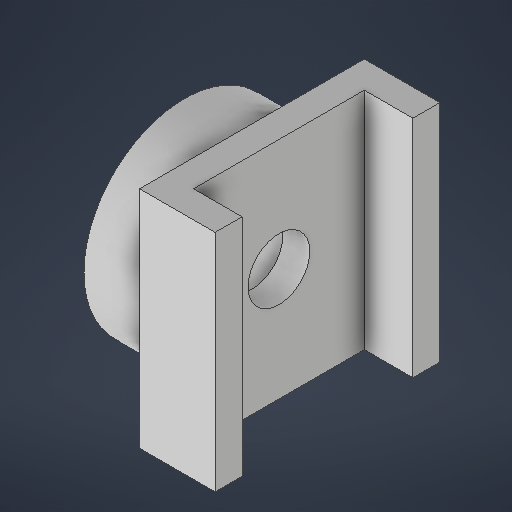
# Autodesk Inventor part: MMAE 232 CAD Assignment 2 Servo Horn 2-Nicholas Skiba
Saved by Autodesk Inventor 2026.1 (Build 301233000, 233)
## iProperties
Created: 2025-08-27
Part Number: MMAE 232 CAD Assignment 2 Servo Horn 2-Nicholas Skiba
Material: Generic
Document SubType Name: Modeling
Designer: Nick
Density: 1 g/cm^3
Appearance: Default
Author: Nick
Autodesk Inventor part; units mm, degrees
ref_plane "YZ Plane" through (0, 0, 0) normal (1, 0, 0) x (0, 1, 0)
ref_plane "XZ Plane" through (0, 0, 0) normal (0, 1, 0) x (-1, 0, 0)
ref_plane "XY Plane" through (0, 0, 0) normal (0, 0, 1) x (1, 0, 0)
sketch "Sketch1" plane through (0, 0, 0) normal (0, 1, 0) x (-1, 0, 0)
  line L0 (0, 0) -> (3.36, 0)
  line L1 (3.36, 0) -> (3.36, -10)
  line L2 (3.36, -10) -> (0, -10)
  line L3 (0, -10) -> (0, -8.8)
  line L4 (0, -8.8) -> (2.16, -8.8)
  line L5 (2.16, -8.8) -> (2.16, -1.2)
  line L6 (2.16, -1.2) -> (0, -1.2)
  line L7 (0, -1.2) -> (0, 0)
  dimension "d0" = 3.36
  dimension "d1" = 10
  dimension "d2" = 1.2
  dimension "d3" = 2.16
  dimension "d4" = 7.6
  constraints: 16 end point, 6 perpendicular, 1 horizontal, 1 point on line, 1 vertical
  measures "d0" distance of L0.start L0.end
  measures "d1" distance of L0.end L1.end
  measures "d2" distance of L2.end L3.end
  measures "d3" distance of L3.end L4.end
  measures "d4" distance of L4.end L5.end
extrude "Extrusion1" add sketch "Sketch1" along normal blind 10
sketch "Sketch2" plane through (-3.36, 0, -10) normal (-1, 0, 0) x (0, 0, 1)
  line L0 (1.2, 0) -> (0, 0) projected
  line L1 (0, 0) -> (0, 5)
  line L2 (0, 5) -> (5, 5)
  circle A0 centre (5, 5) radius 1.37
  circle A1 centre (5, 5) radius 2.75
  circle A2 centre (5, 5) radius 4.475
  point P0 (10, 0)
  dimension "d7" = 5
  dimension "d8" = 5
  dimension "d9" = 2.74
  dimension "d10" = 5.5
  dimension "d11" = 8.95
  constraints: 4 end point, 3 centre point, 3 coincident, 1 perpendicular, 1 vertical
  measures "d7" distance of L0.end L1.end
  measures "d8" distance of L1.end L2.end
  measures "d9" diameter of A0
  measures "d10" diameter of A1
  measures "d11" diameter of A2
extrude "Extrusion2" add sketch "Sketch2" along normal blind 3 contours A2
extrude "Extrusion3" cut sketch "Sketch2" against normal through all contours A0
body "Solid1"
